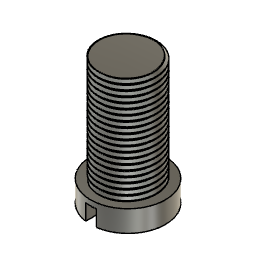
Plattenspielermoebel_Bolzen (Autodesk Fusion 360 design; units mm, degrees)
Autodesk Fusion 360 part; units mm, degrees
note: some values were not read from the file. Chosen so that the rebuilt part matches the saved one: which face or edge a step refers to.
sketch "Skizze1" plane through (0, 0, 0) normal (0, 1, 0) x (1, 0, 0)
  line L0 (0, 0) -> (0, -11)
  line L1 (0, -11) -> (-3.5, -11)
  line L2 (-3.5, -11) -> (-3.5, -10)
  line L3 (-3.5, -10) -> (-2.5, -10)
  line L4 (-2.5, -10) -> (-2.5, 0)
  line L5 (-2.5, 0) -> (0, 0)
  dimension "d1" = 11
  dimension "d2" = 3.5
  dimension "d3" = 1
  dimension "d4" = 1
  constraint coincident L0.start L5.end
  constraint vertical L0
  constraint perpendicular L0 L1
  constraint perpendicular L1 L2
  constraint perpendicular L2 L3
  constraint perpendicular L3 L4
  constraint perpendicular L0 L5
  measures "d1" distance of L0.start L0.end
  measures "d2" distance of L0.end L1.end
  measures "d3" distance of L1.end L2.end
  measures "d4" distance of L2.end L3.end
revolve "Drehen1" add sketch "Skizze1" angle 360 about axis through (0, 0, 0) along (0, 0, 1) makes body 1
sketch "Skizze2" plane through (0, 0, 11) normal (0, 0, 1) x (-1, 0, 0)
  circle A0 centre (0, 0) radius 3.5
  line L0 (0.5, 0) -> (0.5, -3.4641)
  line L1 (-0.5, 0) -> (-0.5, -3.4641)
  line L2 (-0.5, -3.4641) -> (0.5, -3.4641)
  line L3 (0.5, 0) -> (0.5, 3.4641)
  line L4 (-0.5, 0) -> (-0.5, 3.4641)
  line L5 (-0.5, 3.4641) -> (0.5, 3.4641)
  dimension "d6" = 0.5
  dimension "d7" = 0.5
  constraint coincident A0 L0.end
  constraint coincident A0 L1.end
  constraint coincident A0 L3.end
  constraint coincident A0 L4.end
  measures "d6" distance of A0.centre L0.start
  measures "d7" distance of A0.centre L1.start
extrude "Extrusion1" cut sketch "Skizze2" against normal blind 0.5 contours L0 L1 L2 L3 L4 L5 bodies 1
extrude "Extrusion2" cut 1 faces at (-0.0557, -3.4747, 11) along direction (0, 0, -1) blind 0.5 on bodies 1 bodies 1
extrude "Extrusion3" cut 1 faces at (-0.0557, 3.4747, 11) along direction (0, 0, -1) blind 0.5 on bodies 1 bodies 1
mirror "Spiegeln1" about plane through (0, 0, 0) normal (0, 0, -1) of bodies 1 makes body 2
delete_body "Körper entfernen1" bodies 1
move_body "Verschieben1" bodies 2 to x (1, 0, 0) y (0, 1, 0) z (0, 0, 1) at (0, 0, 11)
move_face "Flächen versetzen1" offset 0.3 1 faces at (-2.4969, 0.1246, 4.3333) on bodies 2
extrude "Extrusion4" add 1 faces at (1.9923, 0.7577, 0) along direction (0, 0, -1) blind 1 on bodies 2 bodies 2
extrude "Extrusion5" add 1 faces at (-1.4881, -0.166, 0) along direction (0, 0, -1) blind 1 on bodies 2 bodies 2
thread "Gewinde3" "ISO Metric profile 5.5 M5.5x0.5 6g" major diameter 5.427 minor diameter 4.848 pitch 0.5 angle 60 modelled right hand crest width 0.0671 on face at (-2.7965, 0.1396, 4.3333) crest through (-2.7135, 0, 0.875) on bodies 2
